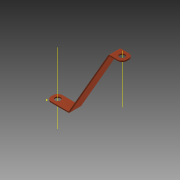
# Autodesk Inventor part: core_earth_new
Saved by Autodesk Inventor 2014 SP1 (Build 180222100, 222)
## iProperties
Created: 2016-11-04
Part Number: core_earth_new
Material: Copper, Cast
Document SubType Name: Sheet Metal
Designer: tguillod
Density: 8.94 g/cm^3
Sheet Metal Rule: Default_mm
Appearance: Copper - Satin
Flat Pattern Width: 0.5 cm
Flat Pattern Length: 5.14236 cm
Flat Pattern Area: 2.57118 cm^2
Sheet Metal Width: 5.000 mm
Sheet Metal Length: 51.424 mm
Sheet Metal Area: 257.118 mm^2
Author: tguillod
Autodesk Inventor part; units mm, degrees
ref_plane "YZ Plane" through (0, 0, 0) normal (1, 0, 0) x (0, 1, 0)
ref_plane "XZ Plane" through (0, 0, 0) normal (0, 1, 0) x (-1, 0, 0)
ref_plane "XY Plane" through (0, 0, 0) normal (0, 0, 1) x (1, 0, 0)
sketch "Sketch1" plane through (0, 0, 0) normal (0, 0, 1) x (1, 0, 0)
  point P0 (0, 0)
sketch "Sketch2" plane through (0, 0, 0) normal (0, 0, 1) x (1, 0, 0)
  line L0 (0, 0) -> (9.852, 0)
  line L1 (9.852, 0) -> (9.852, 5)
  line L2 (9.852, 5) -> (0, 5)
  line L3 (0, 5) -> (0, 0)
  dimension "d0" = 5
  dimension "d1" = 9.852
  measures "d0" distance of L2.end L0.start
  measures "d1" distance of L1.end L2.end
extrude "Plate1" add sketch "Sketch2" along normal blind 0.5
sketch "Sketch3" plane through (9.852, 5, 0.5) normal (0.8660254, 0, -0.5) x (0, 1, 0)
  line L0 (-5, 0) -> (0, 0)
  line L1 (0, 0) -> (0, 35.507)
  line L2 (0, 35.507) -> (-5, 35.507)
  line L3 (-5, 35.507) -> (-5, 0)
  constraints: 6 end point, 1 horizontal, 1 perpendicular, 1 vertical
edge flange "Flange1" height 35.7957 angle 60 thickness 0.5 bend radius 0.5 thickness toward (0.8660254, 0, -0.5) relief tear relief width 0.5 relief depth 0.25 edges at (9.852, 2.5, 0.5) wall of the first edge with corners at (9.852, 0, 0.5) (9.852, 5, 0.5) (27.6055, 5, 31.25) (27.6055, 0, 31.25)
bend "Bend1"
corner "Corner1"
sketch "Sketch4" plane through (28.0385, 0, 31) normal (0, 0, 1) x (1, 0, 0)
  line L0 (0, 5) -> (0, 0)
  line L1 (0, 0) -> (5.7113, 0)
  line L2 (5.7113, 0) -> (5.7113, 5)
  line L3 (5.7113, 5) -> (0, 5)
  constraints: 6 end point, 1 horizontal, 1 perpendicular, 1 vertical
edge flange "Flange2" height 6 angle 60 thickness 0.5 bend radius 0.5 thickness toward (0, 0, 1) relief tear relief width 0.5 relief depth 0.25 edges at (28.0385, 2.5, 31) wall of the first edge with corners at (28.0385, 5, 31) (28.0385, 0, 31) (33.7499, 0, 31) (33.7499, 5, 31)
bend "Bend2"
corner "Corner2"
sketch "Sketch5" plane through (0, 0, 0) normal (0, 0, -1) x (-1, 0, 0)
  line L0 (-9.5633, 5) -> (-9.5633, 0) projected
  line L1 (0, 5) -> (0, 0) projected
  line L2 (0, 2.5) -> (-9.5633, 2.5) construction
  point P0 (-2.5, 2.5)
  dimension "d23" = 2.5
  constraints: 2 end point, 2 midpoint, 1 point on line
  measures "d23" distance from line of L1 point (-2.5, 2.5)
hole "Hole1" at (2.5, 2.5, 0) direction (0, 0, 1) diameter 2.5 depth 0.5 tip angle 118
sketch "Sketch6" plane through (33.7499, 0, 31) normal (0, 0, -1) x (-1, 0, 0)
  line L0 (5.4226, 0) -> (5.4226, 5) projected
  line L1 (0, 5) -> (0, 0) projected
  line L2 (0, 2.5) -> (5.4226, 2.5) construction
  point P0 (33.7498, 0)
  point P1 (2.5, 2.5)
  dimension "d31" = 2.5
  constraints: 2 end point, 2 midpoint, 1 point on line
  measures "d31" distance from line of point (2.5, 2.5) L1
hole "Hole2" at (31.2499, 2.5, 31) direction (0, 0, 1) diameter 2.5 depth 0.5 tip angle 118
fillet "Corner Round1" radius 2 4 edges at (0, 5, 0.25) (0, 0, 0.25) (33.7499, 0, 31.25) (33.7499, 5, 31.25)
equation "\"d29\" = Thickness"
equation "\"d37\" = Thickness"
equation "\"d3\" = BendReliefWidth"
equation "\"d4\" = BendReliefDepth"
equation "\"d5\" = MinimumRemnant"
equation "\"d6\" = BendRadius"
equation "\"d9\" = BendRadius"
equation "\"d10\" = CornerReliefSize"
equation "\"d11\" = GapSize"
equation "\"d12\" = JacobiRadiusSize"
equation "\"d13\" = BendReliefWidth"
equation "\"d14\" = BendReliefDepth"
equation "\"d15\" = MinimumRemnant"
equation "\"d16\" = BendRadius"
equation "\"d19\" = BendRadius"
equation "\"d20\" = CornerReliefSize"
equation "\"d21\" = GapSize"
equation "\"d22\" = JacobiRadiusSize"
equation "\"BendRadius\" = Thickness"
equation "\"BendReliefWidth\" = Thickness"
equation "\"BendReliefDepth\" = 0.5 * Thickness"
equation "\"CornerReliefSize\" = 4 * Thickness"
equation "\"MinimumRemnant\" = 2 * Thickness"
equation "\"TransitionRadius\" = BendRadius"
equation "\"JacobiRadiusSize\" = BendRadius"
equation "\"GapSize\" = Thickness"
equation "\"d2\" = BendRadius"
equation "\"Thickness\" = 0.5"
body "Solid1"
